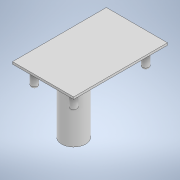
# Autodesk Inventor part: brazo_2_contra
Saved by Autodesk Inventor 2021 (Build 250183000, 183)
## iProperties
Created: 2021-10-12
Part Number: brazo_2_contra
Material: Genérico
Document SubType Name: Modeling
Designer: orgyn
Density: 1 g/cm^3
Appearance: Valor por defecto
Author: orgyn
Autodesk Inventor part; units mm, degrees
ref_plane "YZ Plane" through (0, 0, 0) normal (1, 0, 0) x (0, 1, 0)
ref_plane "XZ Plane" through (0, 0, 0) normal (0, 1, 0) x (-1, 0, 0)
ref_plane "XY Plane" through (0, 0, 0) normal (0, 0, 1) x (1, 0, 0)
sketch "Boceto1" plane through (0, 0, 0) normal (0, 1, 0) x (-1, 0, 0)
  line L0 (0, 0) -> (0, -33)
  line L1 (0, -33) -> (18, -33)
  line L2 (18, -33) -> (18, 0)
  line L3 (18, 0) -> (0, 0)
  circle A0 centre (18, 0) radius 1.5
  circle A1 centre (0, 0) radius 1.5
  circle A2 centre (0, -33) radius 1.5
  circle A3 centre (18, -33) radius 1.5
  line L4 (18, 0) -> (18, 5)
  line L5 (18, 5) -> (23, 5)
  line L6 (23, 5) -> (23, -38)
  line L7 (18, 5) -> (0, 5)
  line L8 (0, 5) -> (-5, 5)
  line L9 (-5, -38) -> (23, -38)
  line L10 (-5, -38) -> (-5, 5)
  line L11 (18, 0) -> (18, -9)
  line L12 (9, -9) -> (18, -9)
  circle A4 centre (9, -9) radius 5.5
  dimension "d0" = 33
  dimension "d1" = 18
  dimension "d2" = 3
  dimension "d3" = 3
  dimension "d4" = 3
  dimension "d5" = 3
  dimension "d6" = 5
  dimension "d7" = 5
  dimension "d8" = 43
  dimension "d9" = 5
  dimension "d10" = 9
  dimension "d11" = 11
  constraints: 26 end point, 7 perpendicular, 5 centre point, 5 coincident, 3 point on line, 1 horizontal, 1 parallel, 1 vertical
  measures "d0" distance of L0.start L0.end
  measures "d1" distance of L0.end L1.end
  measures "d2" diameter of A0
  measures "d3" diameter of A1
  measures "d4" diameter of A2
  measures "d5" diameter of A3
  measures "d6" distance of L4.start L4.end
  measures "d7" distance of L4.end L5.end
  measures "d8" distance of L5.end L6.end
  measures "d9" distance of L7.end L8.end
  measures "d10" distance of L4.start L11.end
  measures "d11" diameter of A4
extrude "Extrusión1" add sketch "Boceto1" along normal blind 3 contours A1 L3 A0 L2 A3 L1 A2 L0 | L5 L6 L9 L10 L8 L7
sketch "Boceto2" plane through (0, 3, 0) normal (0, 1, 0) x (1, 0, 0)
  circle A0 centre (-9, 9) radius 5.5 projected
  circle A1 centre (-9, 9) radius 5.5
  point P0 (0, 0)
  constraints: 1 centre point, 1 coincident
extrude "Extrusión2" add sketch "Boceto2" against normal blind 30
sketch "Boceto3" plane through (0, 3, 0) normal (0, 1, 0) x (1, 0, 0)
  circle A0 centre (0, 0) radius 1.5
  circle A1 centre (-18, 0) radius 1.5 projected
  circle A2 centre (-18, 0) radius 1.5
  circle A3 centre (0, 33) radius 1.5 projected
  circle A4 centre (0, 33) radius 1.5
  circle A5 centre (-18, 33) radius 1.5 projected
  circle A6 centre (-18, 33) radius 1.5
  constraints: 4 centre point, 4 coincident
extrude "Extrusión3" add sketch "Boceto3" against normal blind 10
fillet "Empalme1" radius 1 1 edges at (-19.5, -7, -33)
fillet "Empalme2" radius 1 3 edges at (-19.5, -7, 0) (-1.5, -7, -33) (-1.5, -7, 0)
chamfer "Chaflán1" distance 2 angle 45 4 edges at (-9, 0, -38) (-23, 0, -16.5) (5, 0, -16.5) (-9, 0, 5)
